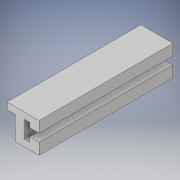
# Autodesk Inventor part: Riel acople de motor
Saved by Autodesk Inventor 2019 (Build 230136000, 136)
## iProperties
Created: 2020-02-02
Part Number: Riel acople de motor
Material: Generic
Document SubType Name: Modeling
Designer: Elías Sánchez
Density: 1 g/cm^3
Appearance: Default
Author: Elías Sánchez
Autodesk Inventor part; units mm, degrees
ref_plane "YZ Plane" through (0, 0, 0) normal (1, 0, 0) x (0, 1, 0)
ref_plane "XZ Plane" through (0, 0, 0) normal (0, 1, 0) x (-1, 0, 0)
ref_plane "XY Plane" through (0, 0, 0) normal (0, 0, 1) x (1, 0, 0)
sketch "Sketch1" plane through (0, 0, 0) normal (0, 0, 1) x (1, 0, 0)
  line L0 (18, 5) -> (18, -3.2)
  line L1 (18, -3.2) -> (11, -3.2)
  line L2 (11, -12.5) -> (11, -9)
  line L3 (11, -9) -> (18, -9)
  line L4 (18, -9) -> (18, -17.5)
  line L5 (18, -17.5) -> (0, -17.5)
  line L6 (0, -17.5) -> (0, 0)
  line L7 (18, 5) -> (-6, 5)
  line L8 (-6, 5) -> (-6, 0)
  line L9 (-6, 0) -> (0, 0)
  line L10 (11, -3.2) -> (11, 0.3)
  line L11 (11, -12.5) -> (7, -12.5)
  line L12 (7, -12.5) -> (7, 0.3)
  line L13 (7, 0.3) -> (11, 0.3)
  dimension "d0" = 6
  dimension "d1" = 5
  dimension "d4" = 4
  dimension "d8" = 5
  dimension "d10" = 5.8
  dimension "d12" = 3.5
  dimension "d13" = 3.5
  dimension "d17" = 0.3
  dimension "d18" = 18
  dimension "d19" = 7
  dimension "d20" = 0
  constraints: 28 end point, 8 perpendicular, 2 horizontal, 2 point on line, 1 vertical
  measures "d0" distance of L8.end L6.end
  measures "d1" distance of L7.end L8.end
  measures "d4" distance between parallel lines of L10 L12
  measures "d8" distance between parallel lines of L5 L11
  measures "d10" distance between parallel lines of L1 L3
  measures "d12" distance of L1.end L10.end
  measures "d13" distance of L2.start L2.end
  measures "d17" distance between parallel lines of L9 L13
  measures "d18" distance between parallel lines of L6 L4
  measures "d19" distance between parallel lines of L6 L12
  measures "d20" distance between parallel lines of L10 L2
extrude "Extrusion1" add sketch "Sketch1" along normal blind 100
equation "\"d13\" = d12"
body "Solid1"
